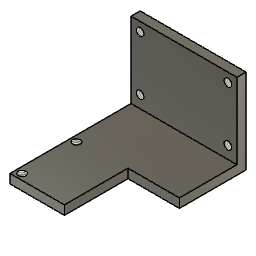
Big Motor Mount v1 (Autodesk Fusion 360 design; units mm, degrees)
Autodesk Fusion 360 part; units mm, degrees
sketch "Sketch1" plane through (0, 0, 0) normal (0, 0, 1) x (1, 0, 0)
  line L0 (0, 0) -> (18, 0)
  line L1 (18, 0) -> (18, 21)
  line L2 (18, 21) -> (0, 21)
  line L3 (0, 21) -> (0, 0)
  line L4 (0, 21) -> (35, 21)
  line L5 (35, 21) -> (35, 43)
  line L6 (35, 43) -> (0, 43)
  line L7 (0, 43) -> (0, 21)
  dimension "d1" = 18
  dimension "d2" = 21
  dimension "d18" = 22
  constraint horizontal L0
  constraint vertical L1
  constraint horizontal L2
  constraint vertical L3
  constraint coincident L0.start L3.end
  constraint horizontal L4
  constraint vertical L5
  constraint horizontal L6
  constraint vertical L7
  measures "d1" distance of L0.start L0.end
  measures "d2" distance of L0.start L2.end
  measures "d18" distance of L2.end L6.end
extrude "Extrude1" add sketch "Sketch1" along normal blind 3
sketch "Sketch2" plane through (0, 0, 3) normal (0, 0, 1) x (-1, 0, 0)
  line L0 (0, -43) -> (0, 0)
  line L1 (0, 0) -> (-18, 0)
  line L2 (-18, 0) -> (-18, -21)
  line L3 (-18, -21) -> (-35, -21)
  line L4 (-35, -21) -> (-35, -43)
  line L5 (-35, -43) -> (0, -43)
  line L6 (0, -43) -> (-35, -43)
  line L7 (-35, -43) -> (-35, -40)
  line L8 (-35, -40) -> (0, -40)
  line L9 (0, -40) -> (0, -43)
  dimension "d5" = 3
  constraint horizontal L6
  constraint vertical L7
  constraint horizontal L8
  constraint vertical L9
  constraint coincident L4 L7.end
  constraint coincident L0.start L5.end
  measures "d5" distance of L0.start L8.end
extrude "Extrude2" add sketch "Sketch2" along normal blind 25 contours L0 L4 L5 L6 L7 L8 L9
sketch "Sketch3" plane through (0, 0, 3) normal (0, 0, 1) x (-1, 0, 0)
  line L0 (-35, -40) -> (0, -40)
  line L1 (0, -40) -> (0, 0)
  line L2 (0, 0) -> (-18, 0)
  line L3 (-18, 0) -> (-18, -21)
  line L4 (-18, -21) -> (-35, -21)
  line L5 (-35, -21) -> (-35, -40)
  circle A0 centre (-2, -2) radius 1.5
  circle A1 centre (-2, -20) radius 1.5
  dimension "d8" = 3
  dimension "d9" = 3
  measures "d8" diameter of A0
  measures "d9" diameter of A1
extrude "Extrude3" cut sketch "Sketch3" against normal blind 4 contours A0 | A1
sketch "Sketch4" plane through (0, 43, 0) normal (0, 1, 0) x (-1, 0, 0)
  line L0 (-35, 0) -> (0, 0)
  line L1 (0, 0) -> (0, 28)
  line L2 (0, 28) -> (-35, 28)
  line L3 (-35, 28) -> (-35, 0)
  circle A0 centre (-32, 25) radius 1.5
  circle A1 centre (-3, 25) radius 1.5
  circle A2 centre (-3, 7) radius 1.5
  circle A3 centre (-32, 7) radius 1.5
  dimension "d12" = 3
  dimension "d13" = 3
  dimension "d14" = 3
  dimension "d15" = 3
  measures "d12" diameter of A0
  measures "d13" diameter of A1
  measures "d14" diameter of A2
  measures "d15" diameter of A3
extrude "Extrude4" cut sketch "Sketch4" against normal blind 4 contours A0 | A1 | A2 | A3
thread "Thread1" "ISO Metric profile 3.0 M3x0.5 6H" major diameter 3.086 minor diameter 2.529 pitch 0.5 angle 60 resizes the face on face at (1.5075, 42, 24.8506)
thread "Thread2" "ISO Metric profile 3.0 M3x0.5 6H" major diameter 3.086 minor diameter 2.529 pitch 0.5 angle 60 resizes the face on face at (1.5075, 42, 6.8506)
thread "Thread3" "ISO Metric profile 3.0 M3x0.5 6H" major diameter 3.086 minor diameter 2.529 pitch 0.5 angle 60 resizes the face on face at (32.6843, 42, 23.6652)
thread "Thread4" "ISO Metric profile 3.0 M3x0.5 6H" major diameter 3.086 minor diameter 2.529 pitch 0.5 angle 60 resizes the face on face at (32.6843, 42, 5.6652)
thread "Thread5" "ISO Metric profile 3.0 M3x0.5 6H" major diameter 3.086 minor diameter 2.529 pitch 0.5 angle 60 resizes the face on face at (0.5075, 20.1494, 2)
thread "Thread6" "ISO Metric profile 3.0 M3x0.5 6H" major diameter 3.086 minor diameter 2.529 pitch 0.5 angle 60 resizes the face on face at (0.5075, 2.1494, 2)
